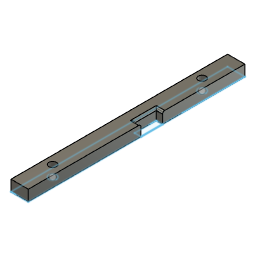
SC126 Base1 v3 (Autodesk Fusion 360 design; units mm, degrees)
Autodesk Fusion 360 part; units mm, degrees
sketch "Sketch1" plane through (0, 0, 0) normal (0, 1, 0) x (1, 0, 0)
  line L0 (0, -29.8938) -> (8, -29.8938)
  line L1 (8, -29.8938) -> (8, 70.1062)
  line L2 (8, 70.1062) -> (0, 70.1062)
  line L3 (0, 70.1062) -> (0, -29.8938)
  circle A0 centre (3.7511, -14.3938) radius 1.75
  circle A1 centre (3.7511, 54.6062) radius 1.75
  line L4 (5.0648, 22.1062) -> (8.0648, 22.1062)
  line L5 (8.0648, 22.1062) -> (8.0648, 32.1062)
  line L6 (8.0648, 32.1062) -> (5.0648, 32.1062)
  line L7 (5.0648, 32.1062) -> (5.0648, 22.1062)
  dimension "d1" = 8
  dimension "d2" = 100
  dimension "d3" = 3.5
  dimension "d4" = 15.5
  dimension "d5" = 3.5
  dimension "d6" = 15.5
  dimension "d7" = 69
  dimension "d10" = 3
  dimension "d11" = 10
  dimension "d16" = 38
  constraint horizontal L0
  constraint vertical L1
  constraint horizontal L2
  constraint vertical L3
  constraint horizontal L4
  constraint vertical L5
  constraint horizontal L6
  constraint vertical L7
  measures "d1" distance of L0.start L0.end
  measures "d2" distance of L0.start L2.end
  measures "d3" diameter of A0
  measures "d4" distance of L0 A0.centre L3.end
  measures "d5" diameter of A1
  measures "d6" distance of L2 A1.centre
  measures "d7" distance of A0.centre A1.centre
  measures "d10" distance of L4.start L4.end
  measures "d11" distance of L4.start L6.end
  measures "d16" distance of L2 L6
extrude "Extrude2" add sketch "Sketch1" along normal blind 5 contours L0 L1 L2 L3 L4 L6 L7
fillet "Fillet1" radius 1 3 edges at (6.5324, 5, -32.1062) (5.0648, 5, -27.1062) (6.5324, 5, -22.1062)
